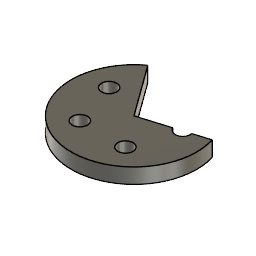
MotorMount_v1 (Autodesk Fusion 360 design; units mm, degrees)
Autodesk Fusion 360 part; units mm, degrees
derive "Sketch8" from "CenterRingV3 v4"
sketch "sketch 220" plane through (0, 0, 6.75) normal (0, 0, 1) x (-1, 0, 0)
  line L0 (3.0331, -7.0669) -> (5.7837, -5.0684)
  line L1 (7.6583, 0.7008) -> (6.6076, 3.9344)
  line L2 (1.7, 7.5) -> (-1.7, 7.5)
  line L3 (-6.6076, 3.9344) -> (-7.6583, 0.7008)
  line L4 (-5.7837, -5.0684) -> (-3.0331, -7.0669)
  circle A0 centre (0, 0) radius 4
  circle A1 centre (0, 0) radius 20
  line L5 (2, 14.4706) -> (2, 21)
  line L6 (-2, 14.4706) -> (-2, 21)
  line L7 (-2, 21) -> (2, 21)
  line L8 (2, 16.5161) -> (-2, 16.5161)
  line L9 (-20.5902, 4.5872) -> (-19.3542, 8.3915)
  line L10 (-14.3804, 2.5696) -> (-20.5902, 4.5872)
  line L11 (-15.0897, 7.0059) -> (-16.3258, 3.2016)
  line L12 (-13.1443, 6.3738) -> (-19.3542, 8.3915)
  line L13 (-10.7255, -18.1649) -> (-13.9615, -15.8138)
  line L14 (-6.8876, -12.8825) -> (-10.7255, -18.1649)
  line L15 (-11.326, -12.1862) -> (-8.0899, -14.5374)
  line L16 (-10.1236, -10.5314) -> (-13.9615, -15.8138)
  line L17 (13.9615, -15.8138) -> (10.7255, -18.1649)
  line L18 (10.1236, -10.5314) -> (13.9615, -15.8138)
  line L19 (8.0899, -14.5374) -> (11.326, -12.1862)
  line L20 (6.8876, -12.8825) -> (10.7255, -18.1649)
  line L21 (19.3542, 8.3915) -> (20.5902, 4.5872)
  line L22 (13.1443, 6.3738) -> (19.3542, 8.3915)
  line L23 (16.3258, 3.2016) -> (15.0897, 7.0059)
  line L24 (14.3804, 2.5696) -> (20.5902, 4.5872)
  line L25 (2, 14.4706) -> (-2, 14.4706)
  line L26 (13.1443, 6.3738) -> (14.3804, 2.5696)
  line L27 (10.1236, -10.5314) -> (6.8876, -12.8825)
  line L28 (-6.8876, -12.8825) -> (-10.1236, -10.5314)
  line L29 (-14.3804, 2.5696) -> (-13.1443, 6.3738)
  line L30 (0, 0) -> (12.3435, -16.9894)
  circle A2 centre (0, 0) radius 16.5161
  line L31 (0, 0) -> (18.9104, -6.5114)
  line L32 (0, 0) -> (12.0363, 15.9727)
  line L33 (0, 0) -> (-11.4715, 16.383)
  line L34 (0, 0) -> (-19.1261, -5.8474)
  line L35 (0, 0) -> (-0.349, -19.997)
  line L36 (4.699, -13.2729) -> (6.5598, -11.921)
  line L37 (14.0753, 0.3675) -> (13.3646, 2.5549)
  line L38 (4, 13.5) -> (1.7, 13.5)
  line L39 (-11.6032, 7.976) -> (-12.3139, 5.7885)
  line L40 (-11.1712, -8.5706) -> (-9.3104, -9.9225)
  line L41 (6.5598, -11.921) -> (3.0331, -7.0669)
  line L42 (5.7837, -5.0684) -> (9.3104, -9.9225)
  line L43 (13.3646, 2.5549) -> (7.6583, 0.7008)
  line L44 (6.6076, 3.9344) -> (12.3139, 5.7885)
  line L45 (1.7, 13.5) -> (1.7, 7.5)
  line L46 (-1.7, 7.5) -> (-1.7, 13.5)
  line L47 (-12.3139, 5.7885) -> (-6.6076, 3.9344)
  line L48 (-7.6583, 0.7008) -> (-13.3646, 2.5549)
  line L49 (-9.3104, -9.9225) -> (-5.7837, -5.0684)
  line L50 (-3.0331, -7.0669) -> (-6.5598, -11.921)
  arc A3 (-8.0902, -4.33) -> (-9.0902, -1.2523) centre (-9.7082, -3.1544) ccw
  line L51 (-8.0902, -4.33) -> (-11.1712, -8.5706)
  line L52 (-6.5598, -11.921) -> (-4.699, -13.2729)
  line L53 (-4.699, -13.2729) -> (-1.618, -9.0322)
  arc A4 (1.618, -9.0322) -> (-1.618, -9.0322) centre (0, -10.2078) ccw
  line L54 (1.618, -9.0322) -> (4.699, -13.2729)
  line L55 (9.3104, -9.9225) -> (11.1712, -8.5706)
  line L56 (11.1712, -8.5706) -> (8.0902, -4.33)
  arc A5 (9.0902, -1.2523) -> (8.0902, -4.33) centre (9.7082, -3.1544) ccw
  line L57 (9.0902, -1.2523) -> (14.0753, 0.3675)
  line L58 (12.3139, 5.7885) -> (11.6032, 7.976)
  line L59 (11.6032, 7.976) -> (6.618, 6.3562)
  arc A6 (4, 8.2583) -> (6.618, 6.3562) centre (6, 8.2583) ccw
  line L60 (4, 8.2583) -> (4, 13.5)
  line L61 (-1.7, 13.5) -> (-4, 13.5)
  line L62 (-4, 13.5) -> (-4, 8.2583)
  arc A7 (-6.618, 6.3562) -> (-4, 8.2583) centre (-6, 8.2583) ccw
  line L63 (-6.618, 6.3562) -> (-11.6032, 7.976)
  line L64 (-13.3646, 2.5549) -> (-14.0753, 0.3675)
  line L65 (-14.0753, 0.3675) -> (-9.0902, -1.2523)
  circle A8 centre (9.7082, -3.1544) radius 2
  circle A9 centre (0, -10.2078) radius 2
  circle A10 centre (-9.7082, -3.1544) radius 2
  circle A11 centre (-6, 8.2583) radius 2
  circle A12 centre (6, 8.2583) radius 2
  circle A13 centre (0, -6) radius 1.25
  circle A14 centre (5.7063, -1.8541) radius 1.25
  circle A15 centre (3.5267, 4.8541) radius 1.25
  circle A16 centre (-3.5267, 4.8541) radius 1.25
  circle A17 centre (-5.7063, -1.8541) radius 1.25
extrude "Extrude1" add sketch "sketch 220" along normal blind 4 contours L0 A0 L30 L31 L42 L55 L56 A5 A8 A14 | L0 L18 L27 L30 A2 L31 L42 L55 L56 A8 | A0 L30 L31 | L18 L27 L30 A2 | A0 L31 L32 | L1 A0 L31 L32 L37 L43 L44 A5 L57 L58 L59 A6 A8 A12 A14 A15 | A0 L32 L33 | A0 L33 L34 | L3 A0 L33 L34 L39 L47 L48 A3 A7 L63 L64 L65 A10 A11 A16 A17 | L31 A14 | L31 A14 | L2 A0 L32 L33 L38 L45 L46 A6 L60 L61 L62 A7 A11 A12 A15 A16 | L34 A17 | L32 A15 | L32 A15 | L33 A16 | L33 A16 | L1 L22 L24 L26 A2 L31 L32 L37 L43 L44 L57 L58 L59 A8 A12 | L22 L24 L26 A2 | L3 L10 L12 L29 A2 L33 L34 L39 L47 L48 L63 L64 L65 A10 A11 | L2 L5 L6 L25 A2 L32 L33 L38 L45 L46 L60 L61 L62 A11 A12 | L10 L12 L29 A2 | L5 L6 L25 A2 picked at (-5.4803, -1.3639)
